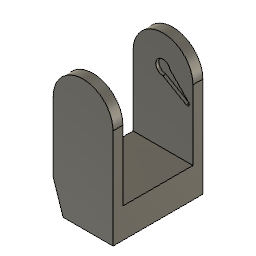
robosoc_leg_holder_V.1 (Autodesk Fusion 360 design; units mm, degrees)
part number: 2025-12-04-10-49-25-755
Autodesk Fusion 360 part; units mm, degrees
sketch "Sketch1" plane through (0, 0, 0) normal (0, 1, 0) x (1, 0, 0)
  line L0 (5, 0) -> (30, 0)
  line L1 (30, 0) -> (30, -50)
  line L2 (0, -50) -> (0, -15)
  arc A0 (0, -50) -> (30, -50) centre (15, -50) ccw
  circle A1 centre (15, -50) radius 1.5
  line L3 (30, 0) -> (5, 0) construction
  line L4 (0, -15) -> (5, 0)
  line L5 (0, -15) -> (30, -15)
  dimension "d2" = 50
  dimension "d4" = 3
  dimension "d5" = 25
  dimension "d6" = 15
  dimension "d9" = 30
  constraint horizontal L0
  constraint vertical L1
  constraint vertical L2
  constraint concentric A0 A1
  constraint perpendicular L1 L3
  constraint perpendicular L1 L5
  measures "d2" distance of origin L2.start
  measures "d4" diameter of A1
  measures "d5" distance of L0.end L0.start
  measures "d6" distance of origin L2.end
  measures "d9" distance of L2.end L5.end
extrude "Extrude1" add sketch "Sketch1" along normal blind 5 contours L0 L1 L4 L5 | L1 L2 A0 L5 | A1
extrude "Extrude2" cut sketch "Sketch1" along normal blind 45 contours L0 L1 L4 L5
extrude "Extrude3" add sketch "Sketch1" along normal blind 22.5 contours L0 L1 L4 L5
mirror "Mirror1" about plane through (0, 22.5, 0) normal (0, 1, 0) of bodies 1 merged
hole "Hole2" at (15, 5, 50) direction (0, -1, 0) diameter 4.5 depth 4 tip angle 180
sketch "Sketch2" plane through (0, 40, 0) normal (0, -1, 0) x (1, 0, 0)
  line L0 (0, 15) -> (30, 15)
  line L1 (30, 15) -> (30, 50)
  arc A0 (30, 50) -> (0, 50) centre (15, 50) ccw
  line L2 (0, 50) -> (0, 15)
  line L3 (14.9863, 46.4) -> (18.4859, 50.8992) construction
  line L4 (15, 50) -> (28.0239, 39.8695) construction
  line L5 (18.4859, 50.8992) -> (27.951, 41.1812)
  line L6 (14.9863, 46.4) -> (26.7346, 39.6174)
  arc A1 (26.7346, 39.6174) -> (27.951, 41.1812) centre (27.2346, 40.4835) ccw
  arc A2 (18.4859, 50.8992) -> (14.9863, 46.4) centre (15, 50) ccw
  dimension "d24" = 7.2
  dimension "d25" = 2
  dimension "d26" = 5.7
  dimension "d28" = 16.5
  constraint concentric A0 A2
  constraint coincident A0.centre L4.start
  constraint coincident L4.end A1
  constraint tangent L5 A1
  constraint tangent L6 A1
  constraint perpendicular L3 L4
  constraint coincident A1.centre L4
  measures "d24" diameter of A2
  measures "d25" diameter of A1
  measures "d26" distance of L3.start L3.end
  measures "d28" distance of A0.centre L4.end
extrude "Extrude4" cut sketch "Sketch2" against normal blind 1.5 contours L5 L6 A1 A2
hole "Hole1" at (17.5, 22.5, 0) direction (0, 0, 1) diameter 19 depth 13 tip angle 180 countersink diameter 21 countersink angle 10
